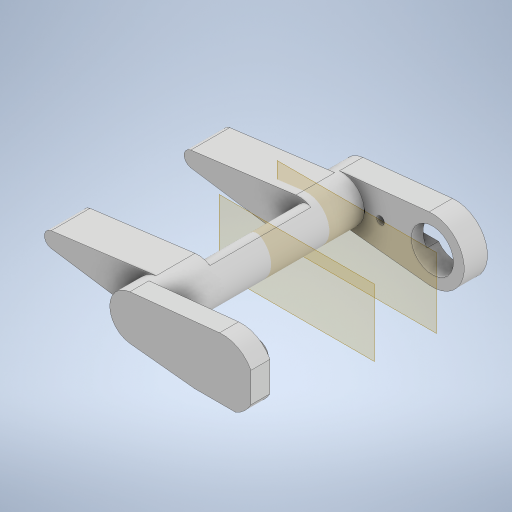
# Autodesk Inventor part: widelec
Saved by Autodesk Inventor 2023 (Build 270158000, 158)
## iProperties
Created: 2023-01-03
Part Number: widelec
Material: Generic
Document SubType Name: Modeling
Designer: Kamil
Density: 1 g/cm^3
Appearance: Default
Author: Kamil
Autodesk Inventor part; units mm, degrees
ref_plane "YZ Plane" through (0, 0, 0) normal (1, 0, 0) x (0, 1, 0)
ref_plane "XZ Plane" through (0, 0, 0) normal (0, 1, 0) x (-1, 0, 0)
ref_plane "XY Plane" through (0, 0, 0) normal (0, 0, 1) x (1, 0, 0)
sketch "Sketch1" plane through (0, 0, 0) normal (0, 0, 1) x (1, 0, 0)
  line L0 (-2.2058, -1.6) -> (-11.675, -1.6) projected
  arc A0 (-2.2058, 1.6) -> (-2.2058, -1.6) centre (0, 0) ccw projected
  line L1 (-11.675, 1.6) -> (-2.2058, 1.6) projected
  arc A1 (-11.675, 1.6) -> (-11.675, -1.6) centre (-11.675, 0) ccw projected
  circle A2 centre (-6.675, 0) radius 0.5 projected
  circle A3 centre (-9.175, 0) radius 0.5 projected
  circle A4 centre (-11.675, 0) radius 0.5 projected
  arc A5 (-2.2058, -1.6) -> (-2.2058, 1.6) centre (0, 0) ccw projected
  line L2 (-2.2058, -1.6) -> (-11.675, -1.6) projected
  arc A6 (-11.675, 1.6) -> (-11.675, -1.6) centre (-11.675, 0) ccw projected
  line L3 (-11.675, 1.6) -> (-2.2058, 1.6) projected
  circle A7 centre (-6.675, 0) radius 0.5 projected
  circle A8 centre (-9.175, 0) radius 0.5 projected
  circle A9 centre (-11.675, 0) radius 0.5 projected
  circle A10 centre (0, 0) radius 1.5 projected
  line L4 (4.125, 1.0232) -> (4.125, -1.0232) projected
  circle A11 centre (0, 0) radius 4.1031
  line L5 (-11.675, 0) -> (-11.675, 4.125)
  circle A12 centre (-11.675, 0) radius 2.9008
  line L6 (-0.4225, 4.0813) -> (-11.9737, 2.8854)
  line L7 (-11.9737, -2.8854) -> (-0.4225, -4.0813)
  constraints: 6 end point, 4 point on circle, 3 coincident, 3 tangent, 2 centre point, 1 vertical
extrude "Extrusion1" add sketch "Sketch1" against normal blind 1.5 contours A5 L1 A11 L0 | A11 L7 A12 L0 | A12 L5 A1 L0 | L1 A12 L5 L6 A11 | L1 L5 A12 | L6 L5 A12
sketch "Sketch2" plane through (0, 0, 0) normal (0, 0, 1) x (1, 0, 0)
  line L0 (-2.2058, -1.6) -> (-11.675, -1.6) projected
  arc A0 (-2.2058, 1.6) -> (-2.2058, -1.6) centre (0, 0) ccw projected
  line L1 (-11.675, 1.6) -> (-2.2058, 1.6) projected
  arc A1 (-11.675, 1.6) -> (-11.675, -1.6) centre (-11.675, 0) ccw projected
  circle A2 centre (-6.675, 0) radius 0.5 projected
  circle A3 centre (-9.175, 0) radius 0.5 projected
  circle A4 centre (-11.675, 0) radius 0.5 projected
  line L2 (-11.9737, -2.8854) -> (-0.4225, -4.0813) projected
  arc A5 (-0.4225, -4.0813) -> (-0.4225, 4.0813) centre (0, 0) ccw projected
  line L3 (-0.4225, 4.0813) -> (-11.9737, 2.8854) projected
  arc A6 (-11.9737, 2.8854) -> (-11.9737, -2.8854) centre (-11.675, 0) ccw projected
  line L4 (-11.675, 1.6) -> (-2.2058, 1.6) projected
  arc A7 (-2.2058, -1.6) -> (-2.2058, 1.6) centre (0, 0) ccw projected
  line L5 (-2.2058, -1.6) -> (-11.675, -1.6) projected
  arc A8 (-11.675, 1.6) -> (-11.675, -1.6) centre (-11.675, 0) ccw projected
  point P0 (-2.2058, 1.6)
extrude "Extrusion2" add sketch "Sketch2" along normal blind 1.5 contours L0 A1 L1 A0 | A6 L3 A5 L2
sketch "Sketch3" plane through (0, 0, 1.5) normal (0, 0, 1) x (1, 0, 0)
  arc A0 (-0.4225, -4.0813) -> (-0.4225, 4.0813) centre (0, 0) ccw projected
  line L0 (-0.4225, 4.0813) -> (-11.9737, 2.8854) projected
  arc A1 (-11.9737, 2.8854) -> (-11.9737, -2.8854) centre (-11.675, 0) ccw projected
  line L1 (-11.9737, -2.8854) -> (-0.4225, -4.0813) projected
  circle A2 centre (-11.675, 0) radius 0.5 projected
  circle A3 centre (-9.175, 0) radius 0.5 projected
  circle A4 centre (-6.675, 0) radius 0.5 projected
  circle A5 centre (0, 0) radius 2.725 projected
  arc A6 (-11.675, 1.6) -> (-11.675, -1.6) centre (-11.675, 0) ccw projected
  circle A7 centre (-11.675, 0) radius 2.9008
  arc A8 (4.0479, -6.2279) -> (4.125, -5.9611) centre (3.625, -5.9611) ccw projected
  line L2 (4.125, -5.9611) -> (4.125, -3.75) projected
  arc A9 (3.625, -4.25) -> (4.125, -3.75) centre (3.625, -3.75) ccw projected
  line L3 (-3.625, -4.25) -> (3.625, -4.25) projected
  arc A10 (-4.125, -3.75) -> (-3.625, -4.25) centre (-3.625, -3.75) ccw projected
  line L4 (-4.125, -3.75) -> (-4.125, -5.9611) projected
  arc A11 (-4.125, -5.9611) -> (-4.0479, -6.2279) centre (-3.625, -5.9611) ccw projected
  arc A12 (-4.0479, -6.2279) -> (-0.925, -7.95) centre (-0.925, -4.2574) ccw projected
  line L5 (-0.925, -7.95) -> (0.925, -7.95) projected
  arc A13 (0.925, -7.95) -> (4.0479, -6.2279) centre (0.925, -4.2574) ccw projected
  circle A14 centre (0, -6.1) radius 0.925 projected
  line L6 (3.625, 15.25) -> (-3.625, 15.25) projected
  line L7 (-3.625, 15.25) -> (-3.625, -3.75) projected
  line L8 (-3.625, -3.75) -> (3.625, -3.75) projected
  line L9 (3.625, -3.75) -> (3.625, 15.25) projected
  circle A15 centre (0, 0) radius 1.9 projected
  arc A16 (4.125, 17.4611) -> (4.0479, 17.7279) centre (3.625, 17.4611) ccw projected
  arc A17 (4.0479, 17.7279) -> (0.925, 19.45) centre (0.925, 15.7574) ccw projected
  line L10 (0.925, 19.45) -> (-0.925, 19.45) projected
  arc A18 (-0.925, 19.45) -> (-4.0479, 17.7279) centre (-0.925, 15.7574) ccw projected
  arc A19 (-4.0479, 17.7279) -> (-4.125, 17.4611) centre (-3.625, 17.4611) ccw projected
  line L11 (-4.125, 17.4611) -> (-4.125, 15.25) projected
  arc A20 (-3.625, 15.75) -> (-4.125, 15.25) centre (-3.625, 15.25) ccw projected
  line L12 (3.625, 15.75) -> (-3.625, 15.75) projected
  arc A21 (4.125, 15.25) -> (3.625, 15.75) centre (3.625, 15.25) ccw projected
  line L13 (4.125, 15.25) -> (4.125, 17.4611) projected
  circle A22 centre (0, 17.6) radius 0.925 projected
  line L14 (-4.125, 15.25) -> (-4.125, -3.75) projected
  line L15 (0, 0) -> (-8, 0)
  dimension "d4" = 8
  constraints: 2 end point, 1 centre point, 1 coincident, 1 horizontal
  measures "d4" distance of L15.start L15.end
extrude "Extrusion3" add sketch "Sketch3" along normal blind 24.55 contours A1 A7 A3 | A3 A7 | A2 picked at (-9.3698, 0.0403)
sketch "Sketch4" plane through (-11.675, 0, 26.05) normal (0, 0, 1) x (1, 0, 0)
  line L0 (15.3, 15.25) -> (8.05, 15.25) projected
  line L1 (8.05, 15.25) -> (8.05, -3.75) projected
  line L2 (8.05, -3.75) -> (15.3, -3.75) projected
  line L3 (15.3, -3.75) -> (15.3, 15.25) projected
  circle A0 centre (11.675, 0) radius 1.9 projected
  circle A1 centre (0, 0) radius 2.9008 projected
  line L4 (11.2525, 4.0813) -> (-0.2987, 2.8854) projected
  line L5 (-0.2987, -2.8854) -> (11.2525, -4.0813) projected
  arc A2 (11.2525, -4.0813) -> (11.2525, 4.0813) centre (11.675, 0) ccw projected
  point P0 (8.0528, -3.75)
  point P1 (13.3401, -3.75)
  point P2 (15.3, -1.9221)
  point P3 (15.3, 1.9221)
extrude "Extrusion4" add sketch "Sketch4" along normal blind 2 contours L3 A2 L2 L1 L4 | L1 L5 A1 L4 | A1 | A0
sketch "Sketch5" plane through (-11.675, 0, 26.05) normal (0, 0, -1) x (-1, 0, 0)
  circle A0 centre (-11.675, 0) radius 1.9 projected
  circle A1 centre (-11.675, 0) radius 1.4377
  point P0 (-11.675, 0)
  constraints: 1 centre point, 1 coincident
extrude "Extrusion5" add sketch "Sketch5" along normal blind 2 contours A1
sketch "Sketch6" plane through (-11.675, 0, 28.05) normal (0, 0, 1) x (1, 0, 0)
  line L0 (-0.2987, -2.8854) -> (8.0528, -3.75) projected
  line L1 (8.0528, -3.75) -> (13.3401, -3.75) projected
  arc A0 (13.3401, -3.75) -> (15.3, -1.9221) centre (11.675, 0) ccw projected
  line L2 (15.3, -1.9221) -> (15.3, 1.9221) projected
  arc A1 (15.3, 1.9221) -> (11.2525, 4.0813) centre (11.675, 0) ccw projected
  line L3 (11.2525, 4.0813) -> (-0.2987, 2.8854) projected
  arc A2 (-0.2987, 2.8854) -> (-0.2987, -2.8854) centre (0, 0) ccw projected
  circle A3 centre (11.675, 0) radius 2.725 projected
  circle A4 centre (5, 0) radius 0.5 projected
  arc A5 (2.8829, 0.3215) -> (-0.2987, 2.8854) centre (0, 0) ccw projected
  arc A6 (2.8829, -0.3215) -> (2.8829, 0.3215) centre (2.5, 0) ccw projected
  arc A7 (-0.2987, -2.8854) -> (2.8829, -0.3215) centre (0, 0) ccw projected
  line L4 (-0.2987, -2.8854) -> (11.2525, -4.0813) projected
  arc A8 (11.2525, -4.0813) -> (11.2525, 4.0813) centre (11.675, 0) ccw projected
  line L5 (11.2525, 4.0813) -> (-0.2987, 2.8854) projected
extrude "Extrusion6" add sketch "Sketch6" along normal blind 0.45 contours A7 A6 A5 L3 A1 L2 A0 L1 L0 | A2 A5 A6 A7 | A3 | A4
ref_plane "Work Plane1" through (-5.4754, 0.1765, 6) normal (0, 0, 1) x (1, 0, 0)
sketch "Sketch7" plane through (-5.4754, 0.1765, 6) normal (0, 0, 1) x (1, 0, 0)
  line L0 (5.0529, -4.2578) -> (-6.4983, -3.0619) projected
  arc A0 (-6.4983, 2.7088) -> (-6.4983, -3.0619) centre (-6.1996, -0.1765) ccw projected
  line L1 (-6.4983, 2.7088) -> (5.0529, 3.9047) projected
  arc A1 (5.0529, -4.2578) -> (5.0529, 3.9047) centre (5.4754, -0.1765) ccw projected
  line L2 (3.2696, 1.4235) -> (-6.1996, 1.4235) projected
  arc A2 (-6.1996, 1.4235) -> (-6.1996, -1.7765) centre (-6.1996, -0.1765) ccw projected
  line L3 (-6.1996, -1.7765) -> (3.2696, -1.7765) projected
  arc A3 (3.2696, -1.7765) -> (3.2696, 1.4235) centre (5.4754, -0.1765) ccw projected
  line L4 (-6.4983, 2.7088) -> (-17.6326, 1.5561)
  line L5 (-17.6326, 1.5561) -> (-17.6326, -1.9092)
  line L6 (-17.6326, -1.9092) -> (-6.4983, -3.0619)
  circle A4 centre (-17.6326, -0.1765) radius 1.7326
  constraints: 6 end point, 1 collinear, 1 midpoint, 1 point on circle, 1 vertical, 3 other
extrude "Extrusion7" add sketch "Sketch7" against normal blind 2 contours L6 A4 L4 A0 | A4 L5 | L5 A4
ref_plane "Work Plane2" through (-11.675, 0, 13.5) normal (0, 0, 1) x (1, 0, 0)
mirror "Mirror1" about plane through (-11.675, 0, 13.5) normal (0, 0, 1) of "Extrusion7"
sketch "Sketch8" plane through (-5.4754, 0.1765, 6) normal (0, 0, 1) x (1, 0, 0)
  line L0 (-6.4983, 2.7088) -> (-17.6326, 1.5561) projected
  arc A0 (-17.6326, 1.5561) -> (-17.6326, -1.9092) centre (-17.6326, -0.1765) ccw projected
  line L1 (-17.6326, -1.9092) -> (-6.4983, -3.0619) projected
  arc A1 (-6.4983, 2.7088) -> (-6.4983, -3.0619) centre (-6.1996, -0.1765) ccw projected
  arc A2 (-6.4983, 2.7088) -> (-6.4983, -3.0619) centre (-6.1996, -0.1765) ccw projected
  arc A3 (-6.4983, 2.7088) -> (-6.4983, -3.0619) centre (-6.1996, -0.1765) ccw projected
  arc A4 (-6.4983, -3.0619) -> (-6.4983, 2.7088) centre (-6.1996, -0.1765) ccw projected
  arc A5 (-6.4983, 2.7088) -> (-6.4983, -3.0619) centre (-6.1996, -0.1765) ccw projected
  arc A6 (-6.4983, 2.7088) -> (-6.4983, -3.0619) centre (-6.1996, -0.1765) ccw projected
  arc A7 (-6.4983, -3.0619) -> (-3.3167, -0.4981) centre (-6.1996, -0.1765) ccw projected
  arc A8 (-3.3167, -0.4981) -> (-3.3167, 0.145) centre (-6.1996, -0.1765) ccw projected
  arc A9 (-3.3167, 0.145) -> (-6.4983, 2.7088) centre (-6.1996, -0.1765) ccw projected
  arc A10 (-6.4983, 2.7088) -> (-6.4983, -3.0619) centre (-6.1996, -0.1765) ccw projected
  arc A11 (-6.4983, 2.7088) -> (-6.4983, -3.0619) centre (-6.1996, -0.1765) ccw projected
  line L2 (-6.4983, 2.7088) -> (-6.4983, -3.0619)
  point P0 (5.4754, -0.1765)
  point P1 (-6.4983, -3.0619)
  constraints: 2 end point, 1 vertical
extrude "Extrusion8" cut sketch "Sketch8" along normal up to surface (15 mm away) contours L2 A1
fillet "Fillet1" radius 1 2 edges at (-11.9737, 2.8854, 13.5) (-11.9737, -2.8854, 13.5)
sketch "Sketch9" plane through (-5.4754, 0.1765, 4) normal (0, 0, -1) x (-1, 0, 0)
  line L0 (17.6326, 1.5561) -> (6.4983, 2.7088) projected
  arc A0 (6.4983, -3.0619) -> (6.4983, 2.7088) centre (6.1996, -0.1765) ccw projected
  line L1 (6.4983, -3.0619) -> (17.6326, -1.9092) projected
  arc A1 (17.6326, -1.9092) -> (17.6326, 1.5561) centre (17.6326, -0.1765) ccw projected
  arc A2 (17.6326, -1.9092) -> (17.6326, 1.5561) centre (17.6326, -0.1765) ccw projected
  line L2 (19.1628, -0.9892) -> (8.9842, -0.9892)
  point P0 (-5.4754, -0.1765)
  constraints: 2 end point, 2 point on circle, 1 horizontal
extrude "Extrusion9" cut sketch "Sketch9" against normal through all contours A1 L1 A0 L2
fillet "Fillet2" radius 1 2 edges at (-24.6382, -0.8127, 22) (-24.6382, -0.8127, 5)
sketch "Sketch10" plane through (-5.4754, 0.1765, 4) normal (0, 0, -1) x (-1, 0, 0)
  arc A0 (18.3409, -0.9892) -> (19.3076, 0.2665) centre (18.3409, 0.0108) ccw projected
  arc A1 (19.3076, 0.2665) -> (17.6326, 1.5561) centre (17.6326, -0.1765) ccw projected
  line L0 (17.6326, 1.5561) -> (6.4983, 2.7088) projected
  arc A2 (8.9842, -0.9892) -> (6.4983, 2.7088) centre (6.1996, -0.1765) ccw projected
  line L1 (8.9842, -0.9892) -> (18.3409, -0.9892) projected
  line L2 (18.3409, -0.9892) -> (18.3409, 0.0108)
  line L3 (18.3409, -0.9892) -> (18.3409, 1.5108)
  arc A3 (19.3076, 0.2665) -> (17.6326, 1.5561) centre (17.6326, -0.1765) ccw projected
  line L4 (18.8714, 1.0349) -> (8.8353, 1.0349)
  line L5 (12.619, 1.0349) -> (12.619, 2.0752)
  line L6 (17.6326, 1.5561) -> (6.4983, 2.7088) projected
  point P0 (-5.4754, -0.1765)
  dimension "d22" = 2.5
  constraints: 8 end point, 3 vertical, 2 point on circle, 2 point on line, 1 horizontal
  measures "d22" distance of L1.end L3.end
extrude "Extrusion10" cut sketch "Sketch10" against normal through all contours L4 L3 A1 | A2 L0 L5 L4 | L4 L5 L0 A1 L3
sketch "Sketch11" plane through (-11.9737, -1.7667, 21) normal (0, 0, -1) x (-1, 0, 0)
  line L0 (12.3731, 2.9781) -> (2.337, 2.9781) projected
  arc A0 (2.337, 2.9781) -> (-1.3689, 4.4628) centre (-0.2987, 1.7667) ccw projected
  arc A1 (0, 3.5334) -> (-1.3689, 4.4628) centre (-1, 3.5334) ccw projected
  line L1 (0, 0) -> (0, 3.5334) projected
  arc A2 (-1.3689, -0.9295) -> (0, 0) centre (-1, 0) ccw projected
  arc A3 (-1.3689, -0.9295) -> (2.4859, 0.954) centre (-0.2987, 1.7667) ccw projected
  line L2 (2.4859, 0.954) -> (11.8426, 0.954) projected
  arc A4 (11.8426, 0.954) -> (12.8093, 2.2097) centre (11.8426, 1.954) ccw projected
  arc A5 (12.8093, 2.2097) -> (12.3731, 2.9781) centre (11.1343, 1.7667) ccw projected
  line L3 (2.4859, 0.954) -> (2.337, 2.9781)
  point P0 (-11.9737, 1.7667)
  constraints: 2 end point
extrude "Extrusion11" add sketch "Sketch11" along normal up to surface (15 mm away) contours L3 A3 A2 L1 A1 A0
sketch "Sketch12" plane through (-14.3107, 1.2114, 21) normal (0, 0, -1) x (-1, 0, 0)
  line L0 (0, 0) -> (10.036, 0) projected
  line L1 (0, 0) -> (0.1489, -2.0241) projected
  line L2 (0.1489, -2.0241) -> (9.5055, -2.0241) projected
  arc A0 (9.5055, -2.0241) -> (10.4723, -0.7684) centre (9.5055, -1.0241) ccw projected
  arc A1 (10.4723, -0.7684) -> (10.036, 0) centre (8.7973, -1.2114) ccw projected
  line L3 (10.036, 0) -> (0, 0) projected
  circle A2 centre (9.5055, -1.0241) radius 1
  line L4 (-13.8882, -5.2926) -> (-2.337, -4.0968) projected
  arc A3 (-2.337, -4.0968) -> (-2.337, 1.674) centre (-2.6357, -1.2114) ccw projected
  line L5 (-2.337, 1.674) -> (-13.8882, 2.8699) projected
  arc A4 (-13.8882, 2.8699) -> (-13.8882, -5.2926) centre (-14.3107, -1.2114) ccw projected
  line L6 (-12.1049, 0.3886) -> (-2.6357, 0.3886) projected
  arc A5 (-2.6357, -2.8114) -> (-2.6357, 0.3886) centre (-2.6357, -1.2114) ccw projected
  line L7 (-2.6357, -2.8114) -> (-12.1049, -2.8114) projected
  arc A6 (-12.1049, 0.3886) -> (-12.1049, -2.8114) centre (-14.3107, -1.2114) ccw projected
  line L8 (11.1552, -1.7515) -> (-1.0983, -3.8879)
  line L9 (8.9077, 0.0714) -> (-1.4688, 1.5522)
  arc A7 (9.5055, -2.0241) -> (10.4723, -0.7684) centre (9.5055, -1.0241) ccw projected
  line L10 (-1.0983, -3.8879) -> (-2.1375, -4.0691)
  line L11 (8.9077, 0.0714) -> (9.408, 0)
  line L12 (10.036, 0) -> (0, 0) projected
  line L13 (-1.4688, 1.5522) -> (-2.2259, 1.6603)
  line L14 (9.408, 0) -> (9.6468, -0.0341)
  point P0 (9.408, 0)
  point P1 (10.4723, -0.7684)
  point P2 (9.6773, -2.0092)
  point P3 (10.4723, -0.7684)
  constraints: 12 end point, 4 tangent, 2 point on circle, 2 point on line, 1 coincident, 6 other
extrude "Extrusion12" cut sketch "Sketch12" against normal blind 4 contours L0 A1 A2 L14
extrude "Extrusion13" add sketch "Sketch12" against normal blind 4 contours A3 L13 L9 L11 L0 | L0 L14 A2 L2 A3 | L2 A0 L8 L10 A3 | A2 A0
sketch "Sketch13" plane through (-5.4754, 0.1765, 6) normal (0, 0, 1) x (1, 0, 0)
  line L0 (-6.6094, 2.6952) -> (-18.4822, 1.0008) projected
  arc A0 (-18.4822, 1.0008) -> (-18.5126, -0.9743) centre (-18.3409, 0.0108) ccw projected
  line L1 (-18.5126, -0.9743) -> (-6.6978, -3.0342) projected
  arc A1 (-6.6094, 2.6952) -> (-6.6978, -3.0342) centre (-6.1996, -0.1765) ccw projected
  line L2 (-8.8353, 1.0349) -> (-8.9842, -0.9892) projected
  arc A2 (-8.9842, -0.9892) -> (-6.6978, -3.0342) centre (-6.1996, -0.1765) ccw projected
  line L3 (-6.6978, -3.0342) -> (-18.5126, -0.9743) projected
  arc A3 (-18.4822, 1.0008) -> (-18.5126, -0.9743) centre (-18.3409, 0.0108) ccw projected
  line L4 (-18.4822, 1.0008) -> (-6.6094, 2.6952) projected
  arc A4 (-6.6094, 2.6952) -> (-8.8353, 1.0349) centre (-6.1996, -0.1765) ccw projected
  line L5 (-8.9842, -0.9892) -> (-8.8353, 1.0349) projected
  line L6 (-8.8353, 1.0349) -> (-18.8714, 1.0349) projected
  arc A5 (-18.8714, 1.0349) -> (-19.3076, 0.2665) centre (-17.6326, -0.1765) ccw projected
  arc A6 (-19.3076, 0.2665) -> (-18.3409, -0.9892) centre (-18.3409, 0.0108) ccw projected
  line L7 (-18.3409, -0.9892) -> (-8.9842, -0.9892) projected
  point P0 (5.4754, -0.1765)
  point P1 (-19.3076, 0.2665)
  point P2 (-18.2433, 1.0349)
extrude "Extrusion14" cut sketch "Sketch13" against normal blind 4 contours L0 A0 A5 L6
extrude "Extrusion15" add sketch "Sketch13" against normal blind 4 contours A1 L6 L0 | L6 A1 L7 A6 A0 L0 | L2 A1 | A1 L1 A6 L7
sketch "Sketch14" plane through (-14.3107, 1.2114, 25) normal (0, 0, 1) x (1, 0, 0)
  line L0 (2.2259, 1.6603) -> (-9.6468, -0.0341) projected
  arc A0 (-9.6468, -0.0341) -> (-9.6773, -2.0092) centre (-9.5055, -1.0241) ccw projected
  line L1 (-9.6773, -2.0092) -> (2.1375, -4.0691) projected
  arc A1 (2.2259, 1.6603) -> (2.1375, -4.0691) centre (2.6357, -1.2114) ccw projected
  line L2 (-9.5055, -1.0241) -> (-3.4186, -1.0241)
  line L3 (2.2259, 1.6603) -> (-9.6468, -0.0341) projected
  line L4 (-7.9977, 0.2013) -> (-7.9977, -2.302)
  line L5 (2.1375, -4.0691) -> (-9.6773, -2.0092) projected
  line L6 (-5.8418, -2.6779) -> (-5.8418, 0.5089)
  circle A2 centre (-7.2024, -1.0596) radius 1.3606
  point P0 (14.3107, -1.2114)
  point P1 (-7.4361, -2.3999)
  point P2 (-7.3946, 0.2873)
  constraints: 6 end point, 4 point on line, 3 tangent, 2 vertical, 1 centre point, 1 horizontal
extrude "Extrusion16" cut sketch "Sketch14" against normal through all contours A2 L4 L0 | L4 A2 L1 A0 L0 | L1 L4 A2
sketch "Sketch15" plane through (-14.3107, 1.2114, 25) normal (0, 0, 1) x (1, 0, 0)
  arc A0 (-7.3946, 0.2873) -> (-7.4361, -2.3999) centre (-7.2024, -1.0596) ccw projected
  line L0 (-7.4361, -2.3999) -> (2.1375, -4.0691) projected
  arc A1 (2.2259, 1.6603) -> (2.1375, -4.0691) centre (2.6357, -1.2114) ccw projected
  line L1 (2.2259, 1.6603) -> (-7.3946, 0.2873) projected
  line L2 (2.1375, -4.0691) -> (-7.4361, -2.3999) projected
  line L3 (-5.0933, -2.8084) -> (-5.0933, 0.6158)
  line L4 (-4.6587, -2.8842) -> (-4.6587, 0.6778)
  line L5 (-7.3946, 0.2873) -> (2.2259, 1.6603) projected
  circle A2 centre (-6.1794, -1.0754) radius 1.5207
  point P0 (14.3107, -1.2114)
  point P1 (-6.4406, -2.5735)
  point P2 (-6.3943, 0.4301)
  constraints: 4 end point, 4 point on line, 3 tangent, 2 vertical, 1 centre point
extrude "Extrusion17" cut sketch "Sketch15" against normal through all contours L1 A2 L0 A0
sketch "Szkic16" plane through (-5.4754, 0.1765, 6) normal (0, 0, 1) x (1, 0, 0)
  arc A0 (-15.2296, 1.4649) -> (-15.276, -1.5386) centre (-15.0148, -0.0405) ccw projected
  line L0 (-15.276, -1.5386) -> (-6.6978, -3.0342) projected
  arc A1 (-8.9842, -0.9892) -> (-6.6978, -3.0342) centre (-6.1996, -0.1765) ccw projected
  line L1 (-8.9842, -0.9892) -> (-8.8353, 1.0349) projected
  arc A2 (-6.6094, 2.6952) -> (-8.8353, 1.0349) centre (-6.1996, -0.1765) ccw projected
  line L2 (-6.6094, 2.6952) -> (-15.2296, 1.4649) projected
  arc A3 (-6.4983, 2.7088) -> (-6.4983, -3.0619) centre (-6.1996, -0.1765) ccw projected
  arc A4 (-6.4983, -3.0619) -> (-6.4983, 2.7088) centre (-6.1996, -0.1765) ccw projected
  arc A5 (-6.4983, 2.7088) -> (-6.4983, -3.0619) centre (-6.1996, -0.1765) ccw projected
  arc A6 (-6.4983, -3.0619) -> (-3.3167, -0.4981) centre (-6.1996, -0.1765) ccw projected
  arc A7 (-3.3167, -0.4981) -> (-3.3167, 0.145) centre (-6.1996, -0.1765) ccw projected
  arc A8 (-3.3167, 0.145) -> (-6.4983, 2.7088) centre (-6.1996, -0.1765) ccw projected
  arc A9 (-8.9842, -0.9892) -> (-6.6978, -3.0342) centre (-6.1996, -0.1765) ccw projected
  arc A10 (-6.6094, 2.6952) -> (-6.6978, -3.0342) centre (-6.1996, -0.1765) ccw projected
  arc A11 (-6.6094, 2.6952) -> (-8.8353, 1.0349) centre (-6.1996, -0.1765) ccw projected
  arc A12 (-6.6094, 2.6952) -> (-8.8353, 1.0349) centre (-6.1996, -0.1765) ccw projected
  arc A13 (-6.6094, 2.6952) -> (-6.6978, -3.0342) centre (-6.1996, -0.1765) ccw projected
  arc A14 (-8.9842, -0.9892) -> (-6.6978, -3.0342) centre (-6.1996, -0.1765) ccw projected
  line L3 (-6.1996, -0.1765) -> (-6.1996, 2.7243)
  line L4 (-6.1996, -0.1765) -> (-6.1996, -3.0773)
  point P0 (5.4754, -0.1765)
  point P1 (-6.4983, -3.0619)
  constraints: 4 end point, 2 point on circle, 1 point on line, 1 vertical
extrude "Wyciągnięcie proste18" cut sketch "Szkic16" along normal up to surface (15 mm away) contours A3 A4 L3 L4 A1 L1 A2
fillet "Zaokrąglenie3" radius 1 2 edges at (-11.675, 2.9008, 13.5) (-11.675, -2.9008, 13.5)
sketch "Szkic17" plane through (-5.4754, 0.1765, 6) normal (0, 0, 1) x (1, 0, 0)
  arc A0 (-15.2296, 1.4649) -> (-15.276, -1.5386) centre (-15.0148, -0.0405) ccw projected
  line L0 (-15.276, -1.5386) -> (-6.6978, -3.0342) projected
  arc A1 (-6.6978, -3.0342) -> (-4.6735, -2.6434) centre (-6.1996, -0.1765) ccw projected
  arc A2 (-6.1996, -1.793) -> (-4.6735, -2.6434) centre (-5.1996, -1.793) ccw projected
  line L1 (-6.1996, -1.793) -> (-6.1996, 1.4399) projected
  arc A3 (-4.6735, 2.2904) -> (-6.1996, 1.4399) centre (-5.1996, 1.4399) ccw projected
  arc A4 (-4.6735, 2.2904) -> (-6.6094, 2.6952) centre (-6.1996, -0.1765) ccw projected
  line L2 (-6.6094, 2.6952) -> (-15.2296, 1.4649) projected
  point P0 (5.4754, -0.1765)
extrude "Wyciągnięcie proste19" cut sketch "Szkic17" against normal blind 0.5
sketch "Szkic18" plane through (-5.4754, 0.1765, 2) normal (0, 0, -1) x (-1, 0, 0)
  arc A0 (15.276, -1.5386) -> (15.2296, 1.4649) centre (15.0148, -0.0405) ccw projected
  circle A1 centre (20.0148, -0.0405) radius 1
  arc A2 (15.276, -1.5386) -> (15.2296, 1.4649) centre (15.0148, -0.0405) ccw projected
  line L0 (15.2296, 1.4649) -> (6.6094, 2.6952) projected
  arc A3 (6.6978, -3.0342) -> (6.6094, 2.6952) centre (6.1996, -0.1765) ccw projected
  line L1 (6.6978, -3.0342) -> (15.276, -1.5386) projected
  line L2 (6.6094, 2.6952) -> (20.1426, 0.9513)
  line L3 (6.6978, -3.0342) -> (20.162, -1.0296)
  point P0 (-5.4754, -0.1765)
  dimension "d44" = 2
  dimension "d45" = 5
  constraints: 4 end point, 2 point on circle, 2 tangent, 1 centre point, 1 horizontal alignment
  measures "d44" diameter of A1
  measures "d45" distance of A1.centre A0.centre
extrude "Wyciągnięcie proste20" add sketch "Szkic18" against normal up to surface (3.5 mm away)
mirror "Odbij2" about plane through (-11.675, 0, 13.5) normal (0, 0, 1) of "Wyciągnięcie proste19", "Wyciągnięcie proste20"
sketch "Szkic19" plane through (-5.4754, 0.1765, 5.5) normal (0, 0, 1) x (1, 0, 0)
  arc A0 (-6.6978, -3.0342) -> (-4.6735, -2.6434) centre (-6.1996, -0.1765) ccw projected
  arc A1 (-6.1996, -1.793) -> (-4.6735, -2.6434) centre (-5.1996, -1.793) ccw projected
  line L0 (-6.1996, 1.4399) -> (-6.1996, -1.793) projected
  arc A2 (-4.6735, 2.2904) -> (-6.1996, 1.4399) centre (-5.1996, 1.4399) ccw projected
  arc A3 (-4.6735, 2.2904) -> (-6.6094, 2.6952) centre (-6.1996, -0.1765) ccw projected
  line L1 (-20.1426, 0.9513) -> (-6.6094, 2.6952) projected
  arc A4 (-20.1426, 0.9513) -> (-20.162, -1.0296) centre (-20.0148, -0.0405) ccw projected
  line L2 (-6.6978, -3.0342) -> (-20.162, -1.0296) projected
  point P0 (5.4754, -0.1765)
extrude "Wyciągnięcie proste21" add sketch "Szkic19" along normal blind 1.5
mirror "Odbij3" about plane through (-11.675, 0, 13.5) normal (0, 0, 1) of "Wyciągnięcie proste21"
body "Solid1"
